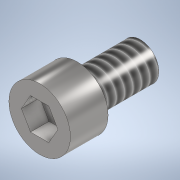
# Autodesk Inventor part: No4_40-3-16
Saved by Autodesk Inventor 2020.4 (Build 244396000, 396)
## iProperties
Created: 2021-09-11
Part Number: No4_40-3-16
Material: ステンレス鋼 AISI 304
Document SubType Name: Modeling
Designer: Masato
Density: 8 g/cm^3
Appearance: 半つや出し
Author: Masato
Autodesk Inventor part; units mm, degrees
ref_plane "YZ Plane" through (0, 0, 0) normal (1, 0, 0) x (0, 1, 0)
ref_plane "XZ Plane" through (0, 0, 0) normal (0, 1, 0) x (-1, 0, 0)
ref_plane "XY Plane" through (0, 0, 0) normal (0, 0, 1) x (1, 0, 0)
sketch "スケッチ1" plane through (0, 0, 0) normal (1, 0, 0) x (0, 1, 0)
  line L0 (0, 7.6073) -> (0, 0)
  line L1 (0, 0) -> (2.3241, 0)
  line L2 (2.3241, 0) -> (2.3241, 2.8448)
  line L3 (2.3241, 2.8448) -> (1.4, 2.8448)
  line L4 (1.4, 2.8448) -> (1.4, 7.6073)
  line L5 (1.4, 7.6073) -> (0, 7.6073)
  dimension "d1" = 1.4
  dimension "d2" = 2.8448
  dimension "d3" = 2.3241
  dimension "d10" = 4.7625
  constraints: 12 end point, 5 perpendicular, 1 vertical
  measures "d1" distance of L0.start L4.end
  measures "d2" distance of L1.end L2.end
  measures "d3" distance of L1.end L0.end
  measures "d10" distance of L3.end L4.end
revolve "回転1" add sketch "スケッチ1" angle 360 about axis through (0, 0, 7.6073) along (0, 0, -1)
sketch "スケッチ2" plane through (0, 0, 0) normal (0, 0, -1) x (-1, 0, 0)
  line L0 (0, 1.3799) -> (1.195, 0.6899)
  line L1 (1.195, 0.6899) -> (1.195, -0.6899)
  line L2 (1.195, -0.6899) -> (0, -1.3799)
  line L3 (0, -1.3799) -> (-1.195, -0.6899)
  line L4 (-1.195, -0.6899) -> (-1.195, 0.6899)
  line L5 (-1.195, 0.6899) -> (0, 1.3799)
  circle A0 centre (0, 0) radius 2.3241 projected
  line L6 (0, 2.3241) -> (0, -2.3241) construction
  point P0 (0, 0)
  dimension "d7" = 2.39
  constraints: 14 end point, 2 point on circle, 1 coincident, 1 midpoint, 1 point on line, 1 vertical, 13 other
  measures "d7" distance between parallel lines of L1 L4
extrude "押し出し1" cut sketch "スケッチ2" against normal blind 1.4 contours L0 L1 L2 L3 L4 L5
thread "ねじ1" size "4-40 UNC" class "2A" standard "ANSI Unified Screw Threads" full length
